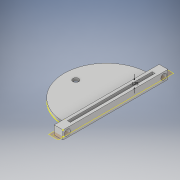
# Autodesk Inventor part: MTV Truning Connecter (10.7)
Saved by Autodesk Inventor 2018 (Build 220112000, 112)
## iProperties
Created: 2018-10-07
Part Number: MTV Truning Connecter (10.7)
Material: Generic
Document SubType Name: Modeling
Designer: Aditya Kendre
Density: 1 g/cm^3
Appearance: Default
Author: Aditya Kendre
Autodesk Inventor part; units mm, degrees
ref_plane "YZ Plane" through (0, 0, 0) normal (1, 0, 0) x (0, 1, 0)
ref_plane "XZ Plane" through (0, 0, 0) normal (0, 1, 0) x (-1, 0, 0)
ref_plane "XY Plane" through (0, 0, 0) normal (0, 0, 1) x (1, 0, 0)
sketch "Sketch1" plane through (0, 0, 0) normal (0, 1, 0) x (-1, 0, 0)
  line L0 (0, 0) -> (9.525, 0)
  line L1 (9.525, 0) -> (9.525, -114.3)
  line L2 (9.525, -114.3) -> (0, -114.3)
  line L3 (0, -114.3) -> (0, 0)
  dimension "d0" = 9.525
  dimension "d1" = 114.3
  constraints: 8 end point, 2 parallel, 1 horizontal, 1 perpendicular
  measures "d0" distance of L1.end L2.end
  measures "d1" distance of L0.end L1.end
extrude "Extrusion1" add sketch "Sketch1" along normal blind 9.525
sketch "Sketch2" plane through (0, 9.525, 0) normal (0, 1, 0) x (1, 0, 0)
  point P0 (0, 0)
sketch "Sketch3" plane through (0, 0, 0) normal (1, 0, 0) x (0, 0, -1)
  circle A0 centre (4.7752, 4.7625) radius 3.175
  circle A1 centre (109.7788, 4.7625) radius 3.175
  point P0 (0, 0)
  dimension "d4" = 6.35
  dimension "d5" = 6.35
  constraints: 2 centre point
  measures "d4" diameter of A0
  measures "d5" diameter of A1
hole "Hole1" at (0, 4.7625, -109.7788) at (0, 4.7625, -4.7752) direction (-1, 0, 0) diameter 6.35 depth 6.35
sketch "Sketch4" plane through (0, 9.525, 0) normal (0, 1, 0) x (1, 0, 0)
  line L0 (-6.35, 106.6038) -> (0, 106.6038) projected
  line L1 (-6.35, 1.6002) -> (-6.35, 7.9502) projected
  line L2 (-3.175, 106.6038) -> (-6.35, 106.6038)
  line L3 (-6.35, 106.6038) -> (-6.35, 7.9502)
  line L4 (-6.35, 7.9502) -> (-3.175, 7.9502)
  line L5 (-3.175, 7.9502) -> (-3.175, 106.6038)
  point P0 (0, 0)
  constraints: 8 end point, 2 parallel, 1 horizontal, 1 midpoint, 1 perpendicular
extrude "Extrusion2" cut sketch "Sketch4" against normal blind 12.7
sketch "Sketch5" plane through (0, 9.525, 0) normal (0, 1, 0) x (1, 0, 0)
  line L0 (-6.35, 106.6038) -> (-6.35, 7.9502) projected
  line L1 (-3.175, 7.9502) -> (-6.35, 7.9502)
  line L2 (-6.35, 7.9502) -> (-6.35, 11.1252)
  line L3 (-6.35, 11.1252) -> (-3.175, 11.1252)
  line L4 (-3.175, 11.1252) -> (-3.175, 7.9502)
  line L5 (-6.35, 106.6038) -> (-3.175, 106.6038) projected
  line L6 (-3.175, 106.6038) -> (-6.35, 106.6038)
  line L7 (-6.35, 106.6038) -> (-6.35, 103.4499)
  line L8 (-6.35, 103.4499) -> (-3.175, 103.4499)
  line L9 (-3.175, 103.4499) -> (-3.175, 106.6038)
  point P0 (0, 0)
  dimension "d15" = 3.175
  constraints: 16 end point, 4 parallel, 2 horizontal, 2 perpendicular, 2 point on line
  measures "d15" distance of L1.end L2.end
extrude "Extrusion3" add sketch "Sketch5" against normal blind 9.525
sketch "Sketch6" plane through (-9.525, 0, -114.3) normal (-1, 0, 0) x (0, 0, 1)
  point P0 (114.3, 0)
sketch "Sketch7" plane through (-9.525, 0, -114.3) normal (-1, 0, 0) x (0, 0, 1)
  line L0 (10.8501, 9.525) -> (10.8501, 0) projected
  line L1 (10.8501, 6.3627) -> (20.6362, 6.3627)
  line L2 (20.6362, 3.1877) -> (10.8501, 3.1877)
  line L3 (10.8501, 3.1877) -> (10.8501, 6.3627)
  line L4 (103.1748, 9.525) -> (103.1748, 0) projected
  line L5 (10.8501, 6.3627) -> (103.1748, 6.3627)
  line L6 (103.1748, 6.3627) -> (103.1748, 3.1877)
  line L7 (103.1748, 3.1877) -> (10.8501, 3.1877)
  line L8 (10.8501, 3.1877) -> (10.8501, 6.3627)
  point P0 (114.3, 0)
  point P1 (10.8501, 4.7625)
  dimension "d18" = 3.175
  constraints: 14 end point, 3 parallel, 2 horizontal, 2 point on line, 1 midpoint, 1 perpendicular
  measures "d18" distance of L1.end L2.start
sketch "Sketch8" plane through (-9.525, 0, -114.3) normal (-1, 0, 0) x (0, 0, 1)
  point P0 (114.3, 0)
ref_plane "Work Plane1" through (-9.525, 3.1877, -11.1252) normal (0, 1, 0) x (0, 0, -1)
sketch "Sketch9" plane through (-9.525, 3.1877, -11.1252) normal (0, 1, 0) x (0, 0, -1)
  point P0 (-11.1252, -9.525)
sketch "Sketch10" plane through (-9.525, 3.1877, -11.1252) normal (0, 1, 0) x (0, 0, -1)
  line L0 (-11.1252, 0) -> (103.1748, 0) projected
  arc A0 (92.2109, 0) -> (0.0002, 0) centre (46.1056, 0.3232) ccw
  line L1 (92.2109, 0) -> (0.0002, 0)
  line L2 (92.3247, -3.175) -> (0, -3.175) projected
  point P0 (-11.1252, -9.525)
  point P1 (-11.1252, -9.525)
  point P2 (-11.1252, -9.525)
  constraints: 2 coincident, 2 end point, 2 point on circle, 2 point on line, 1 centre point, 1 parallel
extrude "Extrusion4" add sketch "Sketch10" along normal blind 3.175
sketch "Sketch11" plane through (-9.525, 3.1877, -11.1252) normal (0, -1, 0) x (1, 0, 0)
  arc A0 (0, -0.0002) -> (0, -92.2109) centre (-0.3232, -46.1056) ccw projected
  line L0 (-46.4297, -46.1056) -> (-33.7222, -46.1056)
  point P0 (9.525, 11.1252)
  constraints: 2 end point, 1 coincident, 1 horizontal, 1 point on circle
sketch "Sketch12" plane through (-9.525, 3.1877, -11.1252) normal (0, -1, 0) x (1, 0, 0)
  point P0 (9.525, 11.1252)
sketch "Sketch13" plane through (-9.525, 3.1877, -11.1252) normal (0, -1, 0) x (1, 0, 0)
  circle A0 centre (-33.7224, -46.1055) radius 3.175
  point P0 (9.525, 11.1252)
  dimension "d22" = 6.35
  constraints: 1 centre point
  measures "d22" diameter of A0
extrude "Extrusion5" cut sketch "Sketch13" against normal blind 3.175
body "Solid1"
